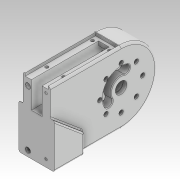
# Autodesk Inventor part: Link2a
Saved by Autodesk Inventor 2020 (Build 240168000, 168)
## iProperties
Created: 2021-03-19
Part Number: Link2a
Material: Generic
Document SubType Name: Modeling
Designer: DDeGo
Density: 1 g/cm^3
Appearance: Default
Author: DDeGo
Autodesk Inventor part; units mm, degrees
ref_plane "YZ Plane" through (0, 0, 0) normal (1, 0, 0) x (0, 1, 0)
sketch "Sketch1" plane through (0, 0, 0) normal (1, 0, 0) x (0, 1, 0)
  line L0 (0, 0) -> (0, -250) construction
  line L1 (-50, 0) -> (-50, -250)
  line L2 (50, -250) -> (50, 0)
  arc A0 (50, 0) -> (-50, 0) centre (0, 0) ccw
  arc A1 (-50, -250) -> (50, -250) centre (0, -250) ccw
  circle A2 centre (0, 0) radius 23.6
  circle A3 centre (0, -250) radius 8.075
  line L3 (50, 0) -> (-50, 0) construction
  point P0 (0, -125)
  dimension "d0" = 50
  dimension "d1" = 250
  dimension "d2" = 47.2
  dimension "d37" = 16.15
  constraints: 10 end point, 4 centre point, 4 point on circle, 4 tangent, 2 coincident, 1 horizontal, 1 midpoint, 1 parallel, 1 vertical
  measures "d0" radius of A0
  measures "d1" distance of L0.start L0.end
  measures "d2" diameter of A2
  measures "d37" diameter of A3
extrude "Extrusion1" add sketch "Sketch1" along normal mid plane 50
sketch "Sketch3" plane through (-25, 50, 0) normal (0, 1, 0) x (1, 0, 0)
  line L0 (0, 300) -> (50, 300) construction
  line L1 (0, 250) -> (50, 250) construction
  line L2 (44, 195) -> (50, 195)
  line L3 (50, 195) -> (50, 305)
  line L4 (50, 305) -> (44, 305)
  line L5 (44, 305) -> (44, 195)
  line L6 (0, 250) -> (50, 250) construction
  line L7 (44, 195) -> (50, 305) construction
  line L8 (50, 195) -> (44, 305) construction
  line L9 (0, 195) -> (6, 195)
  line L10 (6, 195) -> (6, 305)
  line L11 (6, 305) -> (0, 305)
  line L12 (0, 305) -> (0, 195)
  line L13 (0, 195) -> (6, 305) construction
  line L14 (6, 195) -> (0, 305) construction
  line L15 (0, 300) -> (0, 250) construction
  line L16 (50, 250) -> (50, 300) construction
  point P0 (25, 0)
  point P1 (47, 250)
  point P2 (3, 250)
  dimension "d10" = 5
  dimension "d54" = 38
  constraints: 24 end point, 4 collinear, 4 midpoint, 4 parallel, 2 horizontal, 2 perpendicular, 2 point on line
  measures "d10" distance between parallel lines of L4 L0
  measures "d54" distance between parallel lines of L10 L5
extrude "Extrusion3" cut sketch "Sketch3" against normal through all
sketch "Sketch6" plane through (25, 0, 0) normal (1, 0, 0) x (0, 0, -1)
  line L0 (0, 50) -> (195, 50) projected
  line L1 (105.6185, 50) -> (245, 50)
  line L2 (195, -50) -> (195, 50) projected
  line L3 (195, 50) -> (195, -25)
  line L4 (105.6185, 50) -> (195, -25)
  point P0 (0, 0)
  dimension "d21" = 50
  dimension "d22" = 75
  constraints: 6 end point, 1 horizontal, 1 point on line, 2 other
  measures "d21" angle to the sketch y axis of L4
  measures "d22" distance of L3.end L0.end
extrude "Extrusion6" cut sketch "Sketch6" against normal up to surface (6 mm away)
sketch "Sketch7" plane through (-25, 0, 0) normal (-1, 0, 0) x (0, 0, 1)
  line L0 (-250, -50) -> (-195, -50) projected
  arc A0 (-250, 50) -> (-250, -50) centre (-250, 0) ccw projected
  line L1 (-105.6185, 50) -> (-250, 50) projected
  line L2 (-105.6185, 50) -> (-195, -25) projected
  line L3 (-195, -25) -> (-195, -50) projected
  circle A1 centre (-250, 0) radius 8.075 projected
  point P0 (0, 0)
extrude "Extrusion7" cut sketch "Sketch7" against normal up to surface (6 mm away)
sketch "Sketch8" plane through (-25, 50, 0) normal (0, 1, 0) x (1, 0, 0)
  line L0 (30, 50) -> (50, 50)
  line L1 (50, 50) -> (50, -87.0465)
  line L2 (50, -87.0465) -> (30, -87.0465)
  line L3 (30, -87.0465) -> (30, 50)
  line L4 (50, 105.6185) -> (50, 0) projected
  line L5 (0, 0) -> (0, 105.6185) projected
  line L6 (0, 195) -> (0, 0) projected
  line L7 (0, 50) -> (30, 50)
  line L8 (30, 50) -> (30, -87.0465)
  line L9 (30, -87.0465) -> (0, -87.0465)
  line L10 (0, -87.0465) -> (0, 50)
  point P0 (25, 0)
  dimension "d27" = 50
  dimension "d72" = 0
  dimension "d96" = 30
  constraints: 16 end point, 4 parallel, 2 horizontal, 2 perpendicular, 2 point on line, 1 collinear
  measures "d27" distance from line of point (25, 0) L0
  measures "d72" distance between parallel lines of L8 L3
  measures "d96" distance between parallel lines of L5 L3
extrude "Extrusion8" cut sketch "Sketch8" against normal through all contours L0 L1 L2 L3
sketch "Sketch9" plane through (-19, 50, -250) normal (0, 1, 0) x (1, 0, 0)
  line L0 (-6, -144.3815) -> (-6, -55) projected
  line L1 (-6, -55) -> (-6, -58.4641)
  line L2 (-6, -55) -> (0, -55) projected
  line L3 (-6, -58.4641) -> (0, -55)
  line L4 (0, -55) -> (-6, -55)
  line L5 (38, 0) -> (38, -55) projected
  line L6 (44, -55) -> (44, -144.3815) projected
  line L7 (38, -55) -> (44, -55)
  line L8 (44, -55) -> (44, -58.4641)
  line L9 (38, -55) -> (44, -58.4641)
  point P0 (19, -250)
  dimension "d33" = 30
  dimension "d34" = 30
  constraints: 12 end point, 2 point on line, 1 collinear, 1 horizontal
  measures "d33" angle of L7 L9
  measures "d34" angle of L2 L3
extrude "Extrusion9" cut sketch "Sketch9" against normal through all
sketch "Sketch10" plane through (-19, 0, -250) normal (-1, 0, 0) x (0, 0, 1)
  circle A0 centre (0, 0) radius 8.075 projected
  circle A1 centre (0, 0) radius 30 construction
  circle A2 centre (-30, 0) radius 1.65
  circle A3 centre (-21.2132, -21.2132) radius 1.65
  circle A4 centre (0, -30) radius 1.65
  circle A5 centre (21.2132, -21.2132) radius 1.65
  circle A6 centre (30, 0) radius 1.65
  circle A7 centre (21.2132, 21.2132) radius 1.65
  circle A8 centre (0, 30) radius 1.65
  circle A9 centre (-21.2132, 21.2132) radius 1.65
  point P0 (250, 0)
  dimension "d39" = 60
  dimension "d38" = 3.3
  dimension "d42" = 360
  constraints: 8 centre point, 2 horizontal alignment, 1 coincident, 19 other
  measures "d38" diameter of A2
extrude "Extrusion10" cut sketch "Sketch10" against normal through all contours A2 | A3 | A4 | A5 | A6 | A7 | A8 | A9
sketch "Sketch11" plane through (25, 0, 0) normal (1, 0, 0) x (0, 0, -1)
  line L0 (109, -36) -> (151, -36)
  line L1 (151, -36) -> (151, 6)
  line L2 (151, 6) -> (109, 6)
  line L3 (109, 6) -> (109, -36)
  line L4 (109, -36) -> (151, 6) construction
  line L5 (151, -36) -> (109, 6) construction
  circle A0 centre (0, 0) radius 23.6 projected
  point P0 (130, -15)
  dimension "d50" = 42
  dimension "d51" = 42
  dimension "d75" = 15
  dimension "d76" = 130
  constraints: 12 end point, 2 midpoint, 2 parallel, 1 horizontal, 1 perpendicular
  measures "d50" distance of L1.end L2.end
  measures "d51" distance of L0.end L1.end
  measures "d75" vertical distance of A0.centre point (130, -15)
  measures "d76" horizontal distance of point (0, 0) point (130, -15)
extrude "Extrusion11" cut sketch "Sketch11" against normal through all contours L3 L2 L1 L0
sketch "Sketch12" plane through (5, 50, 0) normal (1, 0, 0) x (0, 0, -1)
  circle A0 centre (0, -50) radius 29.5
  circle A1 centre (0, -50) radius 43
  point P0 (0, -50)
  dimension "d55" = 86
  dimension "d56" = 59
  constraints: 2 centre point, 2 coincident
  measures "d55" diameter of A1
  measures "d56" diameter of A0
extrude "Extrusion12" cut sketch "Sketch12" against normal blind 4
ref_plane "Work Plane1" through (-23, 0, 0) normal (-1, 0, 0) x (0, 0, 1)
sketch "Sketch13" plane through (-23, 0, 0) normal (-1, 0, 0) x (0, 0, 1)
  circle A0 centre (0, 0) radius 35
  line L0 (-109, -36) -> (-109, 6) construction
  line L1 (-109, -15) -> (-151, -15) construction
  line L2 (-151, -36) -> (-151, 6) construction
  circle A1 centre (-130, -15) radius 20
  line L3 (-130, -35) -> (0, -35)
  line L4 (-7.9708, 34.0803) -> (-134.5547, 4.4745)
  dimension "d60" = 70
  dimension "d61" = 40
  constraints: 6 end point, 4 point on circle, 4 tangent, 3 midpoint, 2 centre point, 1 coincident
  measures "d60" diameter of A0
  measures "d61" diameter of A1
extrude "Extrusion13" cut sketch "Sketch13" against normal blind 18
sketch "Sketch14" plane through (0, 0, 0) normal (0, 1, 0) x (-1, 0, 0)
  line L0 (5, -23.6) -> (5, 23.6) construction
  line L1 (5, 0) -> (0, 0) construction
  line L2 (-5, -23.6) -> (5, -23.6) construction
  line L3 (-5, 23.6) -> (-5, -23.6) construction
  line L4 (-5, -23.6) -> (-5, -22.1)
  line L5 (-5, -22.1) -> (-2.3, -22.1)
  line L6 (-2.3, -22.1) -> (-2.3, -23.6)
  line L7 (-5, -23.6) -> (-2.3, -23.6)
  dimension "d64" = 1.5
  dimension "d65" = 7.3
  constraints: 10 end point, 2 horizontal, 2 point on line, 1 collinear, 1 midpoint, 1 perpendicular
  measures "d64" distance between parallel lines of L2 L5
  measures "d65" distance between parallel lines of L6 L0
revolve "Revolution1" add sketch "Sketch14" angle 360 about axis through (-5, 0, 0) along (1, 0, 0)
sketch "Sketch15" plane through (-5, 0, 0) normal (-1, 0, 0) x (0, 0, 1)
  line L0 (-109, 6) -> (-151, 6) projected
  line L1 (-109, -36) -> (-109, 6) projected
  line L2 (-151, -36) -> (-109, -36) projected
  line L3 (-151, 6) -> (-151, -36) projected
  line L4 (-109, -36) -> (-151, 6) construction
  circle A0 centre (-130, -15) radius 11
  line L5 (-113, 2) -> (-147, 2) construction
  line L6 (-147, 2) -> (-147, -32) construction
  line L7 (-147, -32) -> (-113, -32) construction
  line L8 (-113, -32) -> (-113, 2) construction
  line L9 (-113, 2) -> (-147, -32) construction
  line L10 (-147, 2) -> (-113, -32) construction
  circle A1 centre (-113, 2) radius 1.75
  circle A2 centre (-113, -32) radius 1.75
  circle A3 centre (-147, -32) radius 1.75
  circle A4 centre (-147, 2) radius 1.75
  point P0 (0, 0)
  dimension "d67" = 22
  dimension "d68" = 34
  dimension "d69" = 3.5
  constraints: 14 end point, 5 centre point, 4 coincident, 3 equal radius, 3 midpoint, 2 parallel, 2 perpendicular, 1 horizontal
  measures "d67" diameter of A0
  measures "d68" distance of L6.end L7.end
  measures "d69" diameter of A2
extrude "Extrusion14" add sketch "Sketch15" against normal blind 3
sketch "Sketch16" plane through (0, 0, 0) normal (1, 0, 0) x (0, 1, 0)
  circle A0 centre (0, -250) radius 8.075 projected
  circle A1 centre (0, -250) radius 40.6397
  line L0 (-19.0139, -214.0826) -> (9, -180.2055)
  line L1 (9, -180.2055) -> (9, -107.6594)
  line L2 (9, -107.6594) -> (-11.0766, -84.8115)
  line L3 (-11.0766, -84.8115) -> (-11.0766, -53.8101)
  line L4 (-11.0766, -53.8101) -> (40.6397, -112.6653)
  line L5 (40.6397, -112.6653) -> (40.6397, -180.2055)
  line L6 (40.6397, -180.2055) -> (37.7306, -234.9007)
  line L7 (40.6397, -180.2055) -> (9, -180.2055) construction
  line L8 (6, -151) -> (6, -109) projected
  point P0 (0, 0)
  dimension "d122" = 3
  constraints: 16 end point, 3 parallel, 2 point on circle, 1 centre point, 1 coincident, 1 perpendicular, 1 vertical
  measures "d122" distance between parallel lines of L1 L8
extrude "Extrusion15" cut sketch "Sketch16" against normal mid plane 15
sketch "Sketch17" plane through (19, 0, -250) normal (1, 0, 0) x (0, 0, -1)
  circle A0 centre (30, 0) radius 1.65 projected
  circle A1 centre (30, 0) radius 3
  circle A2 centre (0, 0) radius 8.075 projected
  circle A3 centre (21.2132, 21.2132) radius 3
  circle A4 centre (0, 30) radius 3
  circle A5 centre (-21.2132, 21.2132) radius 3
  circle A6 centre (-30, 0) radius 3
  circle A7 centre (-21.2132, -21.2132) radius 3
  circle A8 centre (0, -30) radius 3
  circle A9 centre (21.2132, -21.2132) radius 3
  point P0 (-250, 0)
  dimension "d77" = 6
  dimension "d80" = 360
  constraints: 8 centre point, 1 coincident, 17 other
  measures "d77" diameter of A1
extrude "Extrusion16" cut sketch "Sketch17" against normal up to surface (26.5 mm away) contours A0 | A1 | A3 | A4 | A5 | A6 | A7 | A8 | A9
sketch "Sketch18" plane through (0, 0, 0) normal (0, 1, 0) x (-1, 0, 0)
  line L0 (7.5, -258.075) -> (19, -258.075) construction
  line L1 (19, -258.075) -> (19, -241.925) construction
  line L2 (7.5, -241.925) -> (7.5, -258.075) construction
  line L3 (-7.5, -258.075) -> (-7.5, -241.925) construction
  line L4 (-19, -258.075) -> (-7.5, -258.075) construction
  line L5 (-19, -241.925) -> (-19, -258.075) construction
  line L6 (7.5, -250) -> (-19, -250) construction
  line L7 (13.8, -258.075) -> (13.8, -257.075)
  line L8 (13.8, -257.075) -> (-13.8, -257.075)
  line L9 (-13.8, -257.075) -> (-13.8, -258.075)
  line L10 (-19, -258.075) -> (-19, -259.575)
  line L11 (-19, -259.575) -> (19, -259.575)
  line L12 (19, -259.575) -> (19, -258.075)
  line L13 (13.8, -258.075) -> (19, -258.075)
  line L14 (-13.8, -258.075) -> (-19, -258.075)
  point P0 (0, 0)
  dimension "d84" = 5.2
  dimension "d85" = 5.2
  dimension "d86" = 1
  dimension "d87" = 1.5
  constraints: 18 end point, 4 perpendicular, 2 collinear, 2 midpoint, 2 point on line, 2 vertical
  measures "d84" distance between parallel lines of L5 L9
  measures "d85" distance between parallel lines of L1 L7
  measures "d86" distance of L7.start L7.end
  measures "d87" distance between parallel lines of L0 L11
revolve "Revolution2" add sketch "Sketch18" angle 360 about axis through (-7.5, 0, -250) along (1, 0, 0)
sketch "Sketch19" plane through (19, 0, -250) normal (1, 0, 0) x (0, 0, -1)
  circle A0 centre (0, 0) radius 7.075 construction
  arc A1 (6.8404, 18.7939) -> (-17.3205, -10) centre (0, 0) ccw construction
  arc A2 (8.7215, 23.9622) -> (-22.0836, -12.75) centre (0, 0) ccw
  arc A3 (4.9593, 13.6255) -> (-12.5574, -7.25) centre (0, 0) ccw
  arc A4 (4.9593, 13.6255) -> (8.7215, 23.9622) centre (6.8404, 18.7939) ccw
  arc A5 (-22.0836, -12.75) -> (-12.5574, -7.25) centre (-17.3205, -10) ccw
  circle A6 centre (-30, 0) radius 3 projected
  line L0 (0, 0) -> (-30, 0) construction
  line L1 (-17.3205, -10) -> (0, 0) construction
  line L2 (6.8404, 18.7939) -> (0, 0) construction
  point P0 (-250, 0)
  dimension "d89" = 5.5
  dimension "d90" = 20
  dimension "d91" = 30
  dimension "d92" = 110
  constraints: 10 point on circle, 6 end point, 5 centre point, 4 tangent, 1 coincident, 1 horizontal
  measures "d89" radius of A5
  measures "d90" radius of A1
  measures "d91" angle of L0 L1
  measures "d92" angle of L2 L0
extrude "Extrusion17" cut sketch "Sketch19" against normal up to surface (26.5 mm away) contours A4 A3 A5 A2
fillet "Fillet1" radius 50 2 edges at (15, 50, -50) (15, -50, -50)
ref_plane "Work Plane2" through (25, -36, -151) normal (0, 0, 1) x (1, 0, 0)
sketch "Sketch20" plane through (25, -36, -151) normal (0, 0, 1) x (1, 0, 0)
  line L0 (-50, -14) -> (-20, -14) construction
  line L1 (-20, 86) -> (-50, 86) construction
  line L2 (-37.5, -14) -> (-37.5, 86) construction
  circle A0 centre (-37.5, -6) radius 3.2
  circle A1 centre (-37.5, 72) radius 3.2
  point P0 (-25, 36)
  dimension "d98" = 8
  dimension "d99" = 14
  dimension "d100" = 6.4
  dimension "d101" = 12.5
  constraints: 4 point on line, 2 centre point, 2 end point, 1 equal radius, 1 perpendicular
  measures "d98" distance of L2.start A0.centre
  measures "d99" distance of L2.end A1.centre
  measures "d100" diameter of A0
  measures "d101" distance from line of L0.start L2
extrude "Extrusion18" cut sketch "Sketch20" along normal blind 130 and the other way blind 80
sketch "Sketch21" plane through (25, -36, -151) normal (0, 0, 1) x (1, 0, 0)
  line L0 (-44, -14) -> (-6, -14) construction
  line L1 (-44, 86) -> (-6, 86) construction
  line L2 (-12, 86) -> (-12, -14) construction
  circle A0 centre (-12, 76) radius 1.225
  circle A1 centre (-12, -4) radius 1.225
  point P0 (-25, 36)
  dimension "d106" = 2.45
  dimension "d107" = 10
  dimension "d108" = 10
  dimension "d109" = 32
  constraints: 4 point on line, 2 centre point, 2 end point, 1 equal radius, 1 vertical
  measures "d106" diameter of A0
  measures "d107" distance of L2.start A0.centre
  measures "d108" distance of L2.end A1.centre
  measures "d109" distance from line of L1.start L2
extrude "Extrusion19" cut sketch "Sketch21" along normal mid plane 110
sketch "Sketch22" plane through (-19, 50, -250) normal (0, 1, 0) x (1, 0, 0)
  line L0 (3, -1) -> (35, -1)
  line L1 (35, -1) -> (35, -145)
  line L2 (35, -145) -> (3, -145)
  line L3 (3, -145) -> (3, -1)
  line L4 (0, 0) -> (0, -144.3815) projected
  line L5 (38, -144.3815) -> (38, 0) projected
  line L6 (44, -150) -> (24, -150) projected
  line L7 (0, 0) -> (38, 0) projected
  point P0 (19, -250)
  dimension "d112" = 3
  dimension "d113" = 3
  dimension "d114" = 5
  dimension "d115" = 1
  constraints: 8 end point, 2 parallel, 1 horizontal, 1 perpendicular
  measures "d112" distance between parallel lines of L4 L3
  measures "d113" distance between parallel lines of L5 L1
  measures "d114" distance between parallel lines of L6 L2
  measures "d115" distance between parallel lines of L7 L0
extrude "Extrusion20" cut sketch "Sketch22" against normal blind 4
sketch "Sketch23" plane through (-19, 46, -250) normal (0, 1, 0) x (1, 0, 0)
  line L0 (11.5, -5) -> (26.5, -5)
  line L1 (26.5, -5) -> (26.5, -141)
  line L2 (26.5, -141) -> (11.5, -141)
  line L3 (11.5, -141) -> (11.5, -5)
  line L4 (26.5, -69.7945) -> (26.5, -137.3347) projected
  line L5 (11.5, -137.3347) -> (11.5, -69.7945) projected
  line L6 (3, -1) -> (35, -1) projected
  line L7 (35, -145) -> (3, -145) projected
  point P0 (19, -250)
  dimension "d118" = 4
  dimension "d119" = 4
  constraints: 8 end point, 2 parallel, 2 point on line, 1 horizontal, 1 perpendicular
  measures "d118" distance between parallel lines of L6 L0
  measures "d119" distance between parallel lines of L7 L2
extrude "Extrusion21" cut sketch "Sketch23" against normal blind 32.25
sketch "Sketch27" plane through (-25, 0, 0) normal (-1, 0, 0) x (0, 0, 1)
  circle A0 centre (0, 0) radius 30
  dimension "d137" = 60
  constraints: 1 centre point, 1 coincident
  measures "d137" diameter of A0
extrude "Extrusion25" cut sketch "Sketch27" against normal up to surface (2 mm away)
sketch "Sketch24" plane through (-25, 0, 0) normal (-1, 0, 0) x (0, 0, 1)
  circle A0 centre (0, 0) radius 30 projected
  circle A1 centre (0, 0) radius 33
  dimension "d140" = 3
  constraints: 1 centre point, 1 coincident
  measures "d140" radial gap between concentric circles of A1 A0
extrude "Extrusion22" cut sketch "Sketch24" against normal blind 0.5
fillet "Fillet2" radius 3 14 edges at (-19, 0, -300) (-19, -50, -222.5) (-19, 50, -177.8092) (19, 0, -300) (19, -50, -222.5) (19, 50, -177.8092) (-25, 0, 50) (-25, -50, -95.7679) (-25, 50, -52.8092) (25, 0, -50) (25, 50, -102.8092) (25, -50, -145.7679) (22, -50, -193.2679) (-22, -50, -193.2679)
fillet "Fillet3" radius 2 23 edges at (5, 0, -50) (-18.1213, 49.1213, -106.6656) (-19, 11, -152.0968) (-18.1213, -49.1213, -194.4927) (-19, -36, -195) (-22, -23.5466, -193.2679) (-24.1213, 49.1213, -106.6656) (-20.5001, 50, -105.6185) (-17.5001, 50, -105.6185) (17.5001, 50, -105.6185) (20.5001, 50, -105.6185) (-25, 12.4534, -150.3648) (-24.1213, -49.1213, -191.0286) (-25, -34.5467, -191.5359) (18.1213, 49.1213, -106.6656) (19, 11, -152.0968) (24.1213, 49.1213, -106.6656) (25, 12.4534, -150.3648) (22, -23.5466, -193.2679) (18.1213, -49.1213, -194.4927) (19, -36, -195) (24.1213, -49.1213, -191.0286) (25, -34.5467, -191.5359)
sketch "Sketch25" plane through (-19, 46, -250) normal (0, 1, 0) x (1, 0, 0)
  line L0 (7, -137) -> (31, -137) construction
  line L1 (31, -137) -> (31, -9) construction
  line L2 (31, -9) -> (7, -9) construction
  line L3 (7, -9) -> (7, -137) construction
  line L4 (35, -145) -> (3, -145) construction
  line L5 (3, -1) -> (35, -1) construction
  line L6 (3, -144.3815) -> (3, -1) construction
  line L7 (35, -1) -> (35, -144.3815) construction
  circle A0 centre (7, -137) radius 2.15
  circle A1 centre (7, -73) radius 2.15
  circle A2 centre (7, -9) radius 2.15
  circle A3 centre (31, -9) radius 2.15
  line L8 (30.775, -44) -> (30.775, -154) construction
  circle A4 centre (30.775, -73) radius 2.15
  circle A5 centre (31, -137) radius 2.15
  line L9 (7, -73) -> (30.775, -73) construction
  point P0 (19, -250)
  dimension "d128" = 8
  dimension "d129" = 8
  dimension "d130" = 4
  dimension "d131" = 4
  dimension "d132" = 4.3
  constraints: 10 end point, 6 centre point, 5 equal radius, 4 coincident, 2 parallel, 2 perpendicular, 1 horizontal, 1 midpoint, 1 point on line
  measures "d128" distance between parallel lines of L0 L4
  measures "d129" distance between parallel lines of L5 L2
  measures "d130" distance between parallel lines of L6 L3
  measures "d131" distance between parallel lines of L7 L1
  measures "d132" diameter of A0
extrude "Extrusion23" cut sketch "Sketch25" against normal blind 6
sketch "Sketch26" plane through (-25, 0, 0) normal (-1, 0, 0) x (0, 0, 1)
  line L0 (-109, -36) -> (-151, -36) projected
  line L1 (-109, 6) -> (-109, -36) projected
  line L2 (-151, -36) -> (-151, 6) projected
  line L3 (-151, 6) -> (-109, 6) projected
  point P0 (0, 0)
extrude "Extrusion24" add sketch "Sketch26" against normal up to surface (2 mm away)
sketch "Sketch28" plane through (25, 0, 0) normal (1, 0, 0) x (0, 0, -1)
  line L0 (109, -36) -> (109, 6) construction
  line L1 (109, -15) -> (104, -15) construction
  line L2 (99, -5) -> (109, -5)
  line L3 (109, -5) -> (109, -25)
  line L4 (109, -25) -> (99, -25)
  line L5 (99, -25) -> (99, -5)
  line L6 (99, -5) -> (109, -25) construction
  line L7 (109, -5) -> (99, -25) construction
  point P0 (0, 0)
  dimension "d141" = 10
  dimension "d142" = 20
  constraints: 14 end point, 3 midpoint, 2 horizontal, 2 parallel, 1 perpendicular, 1 point on line
  measures "d141" distance of L3.end L4.end
  measures "d142" distance of L4.end L2.start
extrude "Extrusion26" cut sketch "Sketch28" against normal blind 15
sketch "Sketch29" plane through (25, -25, -99) normal (0, 0, -1) x (-1, 0, 0)
  line L0 (0, 0) -> (15, 0) projected
  line L1 (15, 20) -> (7, 20)
  line L2 (7, 20) -> (7, 0)
  line L3 (7, 0) -> (15, 0)
  line L4 (15, 0) -> (15, 20)
  point P0 (25, 25)
  dimension "d145" = 8
  constraints: 8 end point, 2 parallel, 1 horizontal, 1 perpendicular, 1 point on line
  measures "d145" distance between parallel lines of L4 L2
extrude "Extrusion27" cut sketch "Sketch29" against normal blind 23.75
sketch "Sketch30" plane through (10, 0, 0) normal (1, 0, 0) x (0, 0, -1)
  line L0 (109, -25) -> (75.25, -25) projected
  line L1 (99, -5) -> (75.25, -5) projected
  line L2 (75.25, -25) -> (90.25, -25)
  line L3 (90.25, -25) -> (90.25, -5)
  line L4 (90.25, -5) -> (75.25, -5)
  line L5 (75.25, -5) -> (75.25, -25)
  point P0 (0, 0)
  dimension "d148" = 15
  constraints: 8 end point, 2 parallel, 1 horizontal, 1 perpendicular, 1 point on line
  measures "d148" distance between parallel lines of L5 L3
extrude "Extrusion28" cut sketch "Sketch30" against normal up to surface (17.5 mm away)
sketch "Sketch31" plane through (25, -36, -151) normal (0, 0, 1) x (1, 0, 0)
  line L0 (125.1568, -104.5723) -> (-212.9138, -104.5723)
  line L1 (-212.9138, -104.5723) -> (-212.9138, 175.701)
  line L2 (-212.9138, 175.701) -> (125.1568, 175.701)
  line L3 (125.1568, 175.701) -> (125.1568, -104.5723)
  point P0 (-25, 36)
  constraints: 8 end point, 2 parallel, 1 horizontal, 1 perpendicular
extrude "CHOP" cut sketch "Sketch31" along normal through all
sketch "Sketch32" plane through (-19, 0, -250) normal (-1, 0, 0) x (0, 0, 1)
  circle A0 centre (0, 0) radius 8.075 projected
  circle A1 centre (0, 0) radius 38
  circle A2 centre (0, 0) radius 42
  point P0 (250, 0)
  dimension "d153" = 76
  dimension "d154" = 4
  constraints: 2 centre point, 2 coincident
  measures "d153" diameter of A1
  measures "d154" radial gap between concentric circles of A2 A1
extrude "Extrusion30" add sketch "Sketch32" along normal blind 1 contours A2
sketch "Sketch33" plane through (-19, 0, -250) normal (-1, 0, 0) x (0, 0, 1)
  circle A0 centre (21.2132, -21.2132) radius 1.65 construction
  circle A1 centre (0, -30) radius 1.65 construction
  line L0 (21.2132, -21.2132) -> (8.6104, -20.7873) construction
  line L1 (8.6104, -20.7873) -> (0, -30) construction
  line L2 (11.4805, -27.7164) -> (5.7403, -13.8582) construction
  line L3 (13.3283, -26.951) -> (7.588, -13.0928)
  line L4 (3.8925, -14.6236) -> (9.6327, -28.4818)
  arc A2 (9.6327, -28.4818) -> (13.3283, -26.951) centre (11.4805, -27.7164) ccw
  arc A3 (7.588, -13.0928) -> (3.8925, -14.6236) centre (5.7403, -13.8582) ccw
  circle A4 centre (0, 0) radius 7.075 construction
  line L5 (5.7403, -13.8582) -> (0, 0) construction
  point P0 (250, 0)
  dimension "d157" = 22.5
  dimension "d158" = 2
  dimension "d159" = 15
  constraints: 14 end point, 4 point on circle, 4 tangent, 2 centre point, 1 collinear, 1 equal length, 1 midpoint, 1 parallel
  measures "d157" distance of L5.end L0.end
  measures "d158" radius of A2
  measures "d159" distance of L2.start L2.end
extrude "Extrusion31" add sketch "Sketch33" along normal blind 0.8
fillet "Fillet4" radius 0.2 4 edges at (-19.8, -29.5641, -237.7541) (-19.8, -20.0219, -239.5419) (-19.8, -12.0104, -245.0251) (-19.8, -21.5527, -243.2374)
pattern_circular "Circular Pattern1" count 8 over 360 about axis through (0, 0, -250) along (1, 0, 0) of "Extrusion31", "Fillet4"
chamfer "Chamfer1" distance 0.5 angle 45 4 edges at (-15.7, 36, -151) (11.775, 40, -151) (-15.7, -42, -151) (11.775, -40, -151)
fillet "Fillet5" radius 1 8 edges at (7.5, 16.9127, -262.0087) (7.5, 16.3911, -230.4659) (7.5, -14.7631, -235.4295) (7.5, 9.3204, -238.8924) (19, 16.9127, -262.0087) (19, 9.3204, -238.8924) (19, -14.7631, -235.4295) (19, 16.3911, -230.4659)
equation "\"d34\" = d33"
equation "\"d107\" = d108"
equation "\"d113\" = d112"
body "Solid1"
